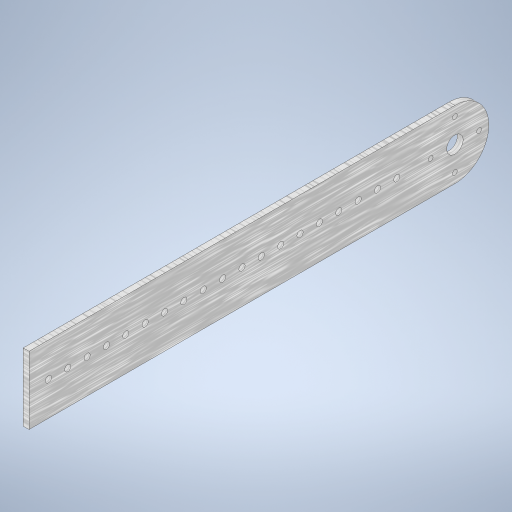
# Autodesk Inventor part: arm_plate1
Saved by Autodesk Inventor 2024 (Build 280153000, 153)
## iProperties
Company: 細田研究室
Created: 2025-06-10
Part Number: arm_plate1
Material: アルミニウム 5052
Document SubType Name: Modeling
Designer: HosodaLab2
Density: 2.68 g/cm^3
Appearance: サテン - ブラシ仕上げ 重厚
個数: 2
Author: HosodaLab2
Autodesk Inventor part; units mm, degrees
ref_plane "YZ Plane" through (0, 0, 0) normal (1, 0, 0) x (0, 1, 0)
ref_plane "XZ Plane" through (0, 0, 0) normal (0, 1, 0) x (-1, 0, 0)
ref_plane "XY Plane" through (0, 0, 0) normal (0, 0, 1) x (1, 0, 0)
sketch "スケッチ1" plane through (0, 0, 0) normal (0, 1, 0) x (-1, 0, 0)
  line L0 (0, 0) -> (-220, 0)
  line L1 (-220, 0) -> (-220, -35)
  line L2 (-220, -35) -> (0, -35)
  line L3 (0, -35) -> (0, 0)
  arc A0 (0, -35) -> (0, 0) centre (0, -17.5) ccw
  dimension "d0" = 220
  dimension "d1" = 35
  dimension "d2" = 17.5
  constraints: 8 end point, 2 parallel, 2 point on circle, 1 centre point, 1 horizontal, 1 perpendicular
  measures "d0" distance of L2.end L1.end
  measures "d1" distance of L1.end L0.end
  measures "d2" radius of A0
extrude "押し出し1" add sketch "スケッチ1" along normal blind 3
sketch "スケッチ2" plane through (0, 3, 0) normal (0, 1, 0) x (1, 0, 0)
  line L0 (0, 17.5) -> (238.6526, 17.5)
  line L1 (0, 0) -> (220, 0) projected
  arc A0 (0, 35) -> (0, 0) centre (0, 17.5) ccw projected
  point P0 (30, 17.5)
  point P1 (40, 17.5)
  point P2 (50, 17.5)
  point P3 (60, 17.5)
  point P4 (70, 17.5)
  point P5 (80, 17.5)
  point P6 (90, 17.5)
  point P7 (100, 17.5)
  point P8 (110, 17.5)
  point P9 (120, 17.5)
  point P10 (130, 17.5)
  point P11 (140, 17.5)
  point P12 (150, 17.5)
  point P13 (160, 17.5)
  point P14 (170, 17.5)
  point P15 (180, 17.5)
  point P16 (190, 17.5)
  point P17 (200, 17.5)
  point P18 (210, 17.5)
  point P19 (-17.5, 17.5)
  dimension "d5" = 17.5
  dimension "d7" = 10
  dimension "d8" = 10
  dimension "d9" = 10
  dimension "d10" = 10
  dimension "d11" = 10
  dimension "d12" = 10
  dimension "d13" = 10
  dimension "d14" = 10
  dimension "d15" = 10
  dimension "d16" = 10
  dimension "d17" = 10
  dimension "d18" = 10
  dimension "d19" = 10
  dimension "d20" = 10
  dimension "d21" = 10
  dimension "d22" = 10
  dimension "d23" = 10
  dimension "d24" = 10
  dimension "d35" = 17.5
  constraints: 1 point on circle, 22 other
  measures "d7" distance of point (40, 17.5) point (30, 17.5)
  measures "d8" distance of point (50, 17.5) point (40, 17.5)
  measures "d9" distance of point (60, 17.5) point (50, 17.5)
  measures "d10" distance of point (70, 17.5) point (60, 17.5)
  measures "d11" distance of point (80, 17.5) point (70, 17.5)
  measures "d12" distance of point (90, 17.5) point (80, 17.5)
  measures "d13" distance of point (100, 17.5) point (90, 17.5)
  measures "d14" distance of point (110, 17.5) point (100, 17.5)
  measures "d15" distance of point (120, 17.5) point (110, 17.5)
  measures "d16" distance of point (130, 17.5) point (120, 17.5)
  measures "d17" distance of point (140, 17.5) point (130, 17.5)
  measures "d18" distance of point (150, 17.5) point (140, 17.5)
  measures "d19" distance of point (160, 17.5) point (150, 17.5)
  measures "d20" distance of point (170, 17.5) point (160, 17.5)
  measures "d21" distance of point (180, 17.5) point (170, 17.5)
  measures "d22" distance of point (190, 17.5) point (180, 17.5)
  measures "d23" distance of point (200, 17.5) point (190, 17.5)
  measures "d24" distance of point (210, 17.5) point (200, 17.5)
  measures "d35" distance of point (-17.5, 17.5) point (0, 17.5)
hole "穴1" at (30, 3, -17.5) at (40, 3, -17.5) at (50, 3, -17.5) at (60, 3, -17.5) at (70, 3, -17.5) at (80, 3, -17.5) at (90, 3, -17.5) at (100, 3, -17.5) at (110, 3, -17.5) at (120, 3, -17.5) at (130, 3, -17.5) at (140, 3, -17.5) at (150, 3, -17.5) at (160, 3, -17.5) at (170, 3, -17.5) at (180, 3, -17.5) at (190, 3, -17.5) at (200, 3, -17.5) at (210, 3, -17.5) direction (0, -1, 0) diameter 3.2 end through all
sketch "スケッチ3" plane through (0, 3, 0) normal (0, 1, 0) x (1, 0, 0)
  line L0 (220, 35) -> (0, 35) projected
  point P0 (0, 0)
  point P1 (0, 17.5)
  dimension "d36" = 17.5
  measures "d36" distance from line of L0 point (0, 17.5)
hole "穴2" at (0, 3, -17.5) direction (0, -1, 0) diameter 8.5 end through all
sketch "スケッチ4" plane through (0, 3, 0) normal (0, 1, 0) x (1, 0, 0)
  circle A0 centre (0, 17.5) radius 12.5
  circle A1 centre (0, 17.5) radius 4.25 projected
  line L0 (-6.6439, 17.5) -> (-13.0454, 17.5)
  line L1 (-13.0454, 17.5) -> (1.0104, 17.5)
  point P0 (0, 0)
  point P1 (0, 5)
  point P2 (12.5, 17.5)
  point P3 (0, 30)
  point P4 (-12.5, 17.5)
  dimension "d44" = 25
  dimension "d45" = 0
  constraints: 4 end point, 4 point on circle, 3 point on line, 1 centre point, 1 horizontal
  measures "d44" diameter of A0
  measures "d45" distance of A0.centre A1.centre
hole "穴3" at (0, 3, -5) at (12.5, 3, -17.5) at (0, 3, -30) at (-12.5, 3, -17.5) direction (0, -1, 0) diameter 2.459 end through all thread size "M3x0.5" class "6H" standard "ISO Metric profile"
